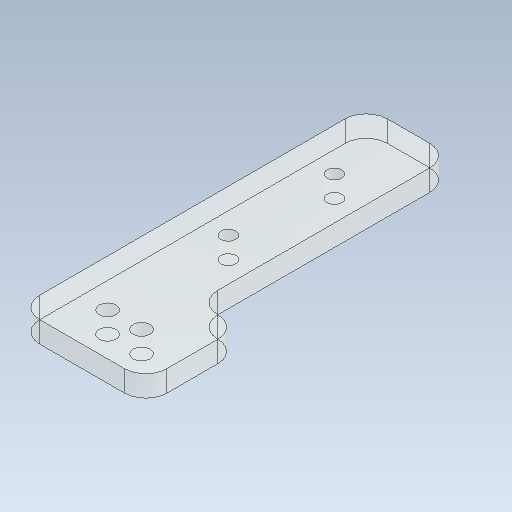
# Autodesk Inventor part: X-Kettenhalter2
Saved by Autodesk Inventor 2021.3 (Build 253353000, 353)
## iProperties
Created: 2021-04-26
Part Number: X-Kettenhalter2
Material: Generic
Document SubType Name: Modeling
Designer: Fabijan_Sven
Density: 1 g/cm^3
Appearance: Clear
Author: Fabijan_Sven
Autodesk Inventor part; units mm, degrees
ref_plane "YZ Plane" through (0, 0, 0) normal (1, 0, 0) x (0, 1, 0)
ref_plane "XZ Plane" through (0, 0, 0) normal (0, 1, 0) x (-1, 0, 0)
ref_plane "XY Plane" through (0, 0, 0) normal (0, 0, 1) x (1, 0, 0)
sketch "Sketch1" plane through (0, 0, 0) normal (0, 1, 0) x (-1, 0, 0)
  line L0 (0, 0) -> (20, 0)
  line L1 (20, 0) -> (20, -82)
  line L2 (20, -82) -> (0, -82)
  line L3 (0, -82) -> (0, 0)
  line L4 (0, 0) -> (-10, 0)
  line L5 (-10, 0) -> (-10, -22)
  line L6 (-10, -22) -> (0, -22)
  line L7 (0, -22) -> (0, 0)
  point P0 (0, -22)
  dimension "d0" = 20
  dimension "d1" = 82
  dimension "d12" = 22
  dimension "d13" = 10
  constraints: 16 end point, 4 parallel, 2 horizontal, 2 perpendicular
  measures "d0" distance of L1.end L2.end
  measures "d1" distance of L0.end L1.end
  measures "d12" distance between parallel lines of L4 L6
  measures "d13" distance between parallel lines of L3 L5
extrude "Extrusion1" add sketch "Sketch1" along normal blind 5
fillet "Fillet1" radius 5 6 edges at (0, 2.5, -82) (-20, 2.5, -82) (-20, 2.5, 0) (10, 2.5, 0) (0, 2.5, -22) (10, 2.5, -22)
sketch "Sketch3" plane through (0, 5, 0) normal (0, 1, 0) x (1, 0, 0)
  line L0 (-24.763, 10) -> (25.9614, 10)
  line L1 (-15, 0) -> (5, 0) projected
  circle A0 centre (-9, 10) radius 2
  circle A1 centre (-1, 10) radius 2
  line L2 (-20, 77) -> (-20, 5) projected
  point P0 (0, 0)
  dimension "d14" = 10
  dimension "d15" = 4
  dimension "d16" = 4
  dimension "d17" = 8
  dimension "d18" = 11
  constraints: 2 centre point, 2 end point, 2 point on line, 1 horizontal
  measures "d14" distance between parallel lines of L1 L0
  measures "d15" diameter of A0
  measures "d16" diameter of A1
  measures "d17" distance of A1.centre A0.centre
  measures "d18" distance from line of L2 A0.centre
hole "Hole2" at (-9, 5, -10) at (-1, 5, -10) direction (0, -1, 0) diameter 4 end through all
sketch "Sketch4" plane through (0, 5, 0) normal (0, 1, 0) x (1, 0, 0)
  circle A0 centre (-10, 64.5) radius 1.5 projected
  circle A1 centre (-10, 39.5) radius 1.5 projected
  point P0 (0, 0)
hole "Hole3" at (-10, 5, -64.5) at (-10, 5, -39.5) direction (0, -1, 0) diameter 3.5 end through all
equation "\"d16\" = d15"
equation "\"d19\" = d15"
body "Solid1"
